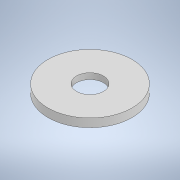
# Autodesk Inventor part: Крышка сальников
Saved by Autodesk Inventor 2021 (Build 250183000, 183)
## iProperties
Created: 2020-11-05
Part Number: Крышка сальников
Material: Типовые
Document SubType Name: Modeling
Designer: Тимоха
Density: 1 g/cm^3
Appearance: По умолчанию
Author: Тимоха
Autodesk Inventor part; units mm, degrees
ref_plane "YZ Plane" through (0, 0, 0) normal (1, 0, 0) x (0, 1, 0)
ref_plane "XZ Plane" through (0, 0, 0) normal (0, 1, 0) x (-1, 0, 0)
ref_plane "XY Plane" through (0, 0, 0) normal (0, 0, 1) x (1, 0, 0)
sketch "Эскиз1" plane through (0, 0, 0) normal (0, 0, 1) x (1, 0, 0)
  line L0 (0, 0) -> (0, 18)
  line L1 (0, 18) -> (100, 18)
  line L2 (100, 18) -> (100, -2)
  line L3 (100, -2) -> (70, -2)
  line L4 (70, -2) -> (70, -8)
  line L5 (70, -8) -> (50, -8)
  line L6 (50, -8) -> (50, 4)
  line L7 (50, 4) -> (32, 4)
  line L8 (32, 4) -> (32, 18)
  dimension "d7" = 18
  dimension "d8" = 100
  dimension "d9" = 20
  dimension "d10" = 30
  dimension "d11" = 20
  dimension "d12" = 12
  dimension "d13" = 18
  constraints: 18 end point, 6 perpendicular, 2 vertical, 1 horizontal, 1 point on line
  measures "d7" distance of L0.start L0.end
  measures "d8" distance of L0.end L1.end
  measures "d9" distance of L1.end L2.end
  measures "d10" distance of L2.end L3.end
  measures "d11" distance of L4.end L5.end
  measures "d12" distance of L5.end L6.end
  measures "d13" distance of L6.end L7.end
revolve "Вращение1" add sketch "Эскиз1" angle 360 about axis through (0, 0, 0) along (0, 1, 0)
